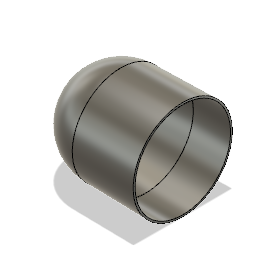
nose01 (Autodesk Fusion 360 design; units mm, degrees)
Autodesk Fusion 360 part; units mm, degrees
sketch "スケッチ1" plane through (0, 0, 0) normal (0, 0, 1) x (1, 0, 0)
  arc A0 (13.6, 12) -> (1.6, 0) centre (13.6, 0) ccw
  line L0 (13.6, 0) -> (13.6, 12) construction
  line L1 (13.6, 0) -> (1.6, 0) construction
  arc A1 (13.6, 13.6) -> (0, 0) centre (13.6, 0) ccw
  line L2 (13.6, 0) -> (13.6, 13.6) construction
  line L3 (13.6, 0) -> (0, 0) construction
  line L4 (0, 0) -> (1.6, 0)
  line L5 (13.6, 13.6) -> (30, 13.6)
  line L6 (30, 13.6) -> (30, 12.8)
  line L7 (30, 12.8) -> (20, 12.8)
  line L8 (20, 12.8) -> (20, 12)
  line L9 (20, 12) -> (13.6, 12)
  line L10 (1.6, 0) -> (0.6, 0)
  circle A2 centre (13.6, 0) radius 13
  line L11 (20, 12.8) -> (12.2519, 11.924)
  line L12 (30, 12.8) -> (30, 13.3)
  line L13 (30, 13.3) -> (13.3639, 12.9979)
  dimension "d1" = 90
  dimension "d2" = 90
  dimension "d4" = 1
  dimension "d5" = 0.5
  measures "d1" angle of L0 L1
  measures "d2" angle of L2 L3
  measures "d4" distance of A1.end
revolve "回転2" add sketch "スケッチ1" angle 360 about axis through (13.6, 0, 0) along (-1, 0, 0) contours A0 L4 L10 A2 L11 | L6 L7 A2 L11 L12 L13
revolve "回転1" [suppressed]
